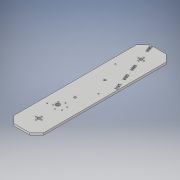
# Autodesk Inventor part: testPart_chassis2
Saved by Autodesk Inventor 2019 (Build 230136000, 136)
## iProperties
Created: 2019-09-17
Part Number: testPart_chassis2
Material: Generic
Document SubType Name: Modeling
Designer: shrey
Density: 1 g/cm^3
Appearance: Default
Author: shrey
Autodesk Inventor part; units mm, degrees
ref_plane "YZ Plane" through (0, 0, 0) normal (1, 0, 0) x (0, 1, 0)
ref_plane "XZ Plane" through (0, 0, 0) normal (0, 1, 0) x (-1, 0, 0)
ref_plane "XY Plane" through (0, 0, 0) normal (0, 0, 1) x (1, 0, 0)
sketch "Sketch1" plane through (0, 0, 0) normal (0, 1, 0) x (-1, 0, 0)
  line L0 (-44.45, -203.2) -> (44.45, -203.2)
  line L1 (44.45, -203.2) -> (44.45, 203.2)
  line L2 (44.45, 203.2) -> (-44.45, 203.2)
  line L3 (-44.45, 203.2) -> (-44.45, -203.2)
  line L4 (-44.45, -203.2) -> (44.45, 203.2) construction
  line L5 (44.45, -203.2) -> (-44.45, 203.2) construction
  line L6 (0, 203.2) -> (0, -203.2) construction
  line L7 (0, 0) -> (44.45, 0) construction
  line L8 (0, -203.2) -> (0, 203.2) construction
  line L9 (0, 152.4) -> (7.112, 152.4) construction
  line L10 (0, -152.4) -> (0, -203.2) construction
  circle A0 centre (0, -152.4) radius 8 construction
  line L11 (0, 152.4) -> (-44.45, 152.4) construction
  line L12 (-44.45, 152.4) -> (-44.45, 88.9)
  line L13 (-44.45, 88.9) -> (0, 88.9) construction
  line L14 (0, 88.9) -> (0, 152.4) construction
  circle A1 centre (0, 88.9) radius 7.112 construction
  circle A2 centre (7.112, 88.9) radius 5.9944
  circle A3 centre (0, 88.9) radius 15.494 construction
  circle A4 centre (0, 104.394) radius 1.5
  circle A5 centre (0, 88.9) radius 15.494 construction
  circle A6 centre (-13.4182, 96.647) radius 1.5
  circle A7 centre (0, 88.9) radius 15.494 construction
  circle A8 centre (-13.4182, 81.153) radius 1.5
  circle A9 centre (0, 88.9) radius 15.494 construction
  circle A10 centre (0, 73.406) radius 1.5
  circle A11 centre (0, 88.9) radius 15.494 construction
  circle A12 centre (13.4182, 81.153) radius 1.5
  circle A13 centre (0, 88.9) radius 15.494 construction
  circle A14 centre (13.4182, 96.647) radius 1.5
  circle A15 centre (0, 152.4) radius 4
  circle A16 centre (0, 152.4) radius 8 construction
  circle A17 centre (0, 160.4) radius 1.85
  circle A18 centre (0, 152.4) radius 8 construction
  circle A19 centre (-8, 152.4) radius 1.85
  circle A20 centre (0, 152.4) radius 8 construction
  circle A21 centre (0, 144.4) radius 1.85
  circle A22 centre (0, 152.4) radius 8 construction
  circle A23 centre (8, 152.4) radius 1.85
  line L15 (-88.9, 44.45) -> (0, 44.45) construction
  line L16 (0, 44.45) -> (0, -44.45) construction
  line L17 (0, -44.45) -> (-88.9, -44.45) construction
  line L18 (-88.9, -44.45) -> (-88.9, 44.45) construction
  line L19 (-88.9, 44.45) -> (0, -44.45) construction
  line L20 (0, 44.45) -> (-88.9, -44.45) construction
  circle A24 centre (0, 44.45) radius 2.9766
  circle A25 centre (0, -44.45) radius 2.9766
  line L21 (44.45, -203.2) -> (25.4, -203.2)
  line L22 (25.4, -203.2) -> (25.4, -101.6) construction
  line L23 (25.4, -101.6) -> (44.45, -101.6) construction
  line L24 (44.45, -101.6) -> (44.45, -203.2)
  circle A26 centre (25.9021, -101.6) radius 1.5875
  circle A27 centre (25.9021, 101.6) radius 1.5875
  line L25 (-44.45, 0) -> (-22.225, 0)
  line L26 (-44.45, -17.5714) -> (-25.4, -17.5714) construction
  line L27 (-25.4, -17.5714) -> (-25.4, 31.4423) construction
  line L28 (-25.4, 31.4423) -> (-44.45, 31.4423) construction
  line L29 (-44.45, 31.4423) -> (-44.45, -17.5714)
  circle A28 centre (-25.4, 0) radius 1.5875
  line L30 (-44.45, -203.2) -> (0, -203.2)
  line L31 (0, 0) -> (-44.45, 0)
  line L32 (-44.45, 0) -> (-44.45, -203.2)
  line L33 (-44.45, -203.2) -> (19.05, -203.2)
  line L34 (19.05, -203.2) -> (19.05, -25.4) construction
  line L35 (19.05, -25.4) -> (-44.45, -25.4) construction
  line L36 (-44.45, -25.4) -> (-44.45, -203.2)
  line L37 (19.05, -203.2) -> (-44.45, -25.4) construction
  line L38 (-44.45, -25.4) -> (-38.0428, -43.3402) construction
  line L39 (-30.3832, -55.3489) -> (-36.3634, -57.4842)
  line L40 (-36.3634, -57.4842) -> (-42.7694, -39.5436)
  line L41 (-42.7694, -39.5436) -> (-36.7892, -37.4083)
  line L42 (-36.7892, -37.4083) -> (-30.3832, -55.3489)
  line L43 (-41.2178, -33.8152) -> (-34.8678, -52.8652) construction
  line L44 (-34.8678, -33.8152) -> (-41.2178, -52.8652) construction
  line L45 (-23.549, -93.3646) -> (-29.955, -75.424)
  line L46 (-17.5688, -91.2293) -> (-23.549, -93.3646)
  line L47 (-23.9748, -73.2887) -> (-17.5688, -91.2293)
  line L48 (-29.955, -75.424) -> (-23.9748, -73.2887)
  line L49 (-10.7346, -129.245) -> (-17.1406, -111.3044)
  line L50 (-4.7544, -127.1096) -> (-10.7346, -129.245)
  line L51 (-11.1604, -109.169) -> (-4.7544, -127.1096)
  line L52 (-17.1406, -111.3044) -> (-11.1604, -109.169)
  line L53 (2.0798, -165.1253) -> (-4.3262, -147.1847)
  line L54 (8.06, -162.99) -> (2.0798, -165.1253)
  line L55 (1.654, -145.0494) -> (8.06, -162.99)
  line L56 (-4.3262, -147.1847) -> (1.654, -145.0494)
  line L57 (14.8942, -201.0057) -> (8.4882, -183.0651)
  line L58 (20.8744, -198.8704) -> (14.8942, -201.0057)
  line L59 (14.4684, -180.9298) -> (20.8744, -198.8704)
  line L60 (8.4882, -183.0651) -> (14.4684, -180.9298)
  circle A29 centre (0, -152.4) radius 4
  circle A30 centre (0, -160.4) radius 1.85
  circle A31 centre (-8, -152.4) radius 1.85
  circle A32 centre (0, -144.4) radius 1.85
  circle A33 centre (8, -152.4) radius 1.85
  dimension "d26" = 14.224
  dimension "d28" = 30.988
  dimension "d40" = 16
  dimension "d0" = 406.4
  dimension "d1" = 88.9
  dimension "d2" = 152.4
  dimension "d17" = 16
  dimension "d24" = 44.45
  dimension "d25" = 63.5
  dimension "d27" = 11.9888
  dimension "d29" = 3
  dimension "d32" = 360
  dimension "d39" = 8
  dimension "d41" = 3.7
  dimension "d44" = 360
  dimension "d63" = 88.9
  dimension "d64" = 5.9531
  dimension "d65" = 5.9531
  dimension "d71" = 101.6
  dimension "d72" = 19.05
  dimension "d73" = 3.175
  dimension "d74" = 19.05
  dimension "d75" = 3.175
  dimension "d81" = 177.8
  dimension "d82" = 63.5
  dimension "d83" = 19.05
  dimension "d84" = 6.35
  dimension "d85" = 19.05
  dimension "d88" = 38.1
  constraints: 122 end point, 23 centre point, 15 parallel, 10 midpoint, 9 coincident, 9 horizontal, 9 point on line, 9 symmetric about line, 7 perpendicular, 4 vertical alignment, 3 horizontal alignment, 1 collinear, 105 other
  measures "d0" distance of L0.end L1.end
  measures "d1" distance of L1.end L2.end
  measures "d2" distance of L7.start point (0, 152.4)
  measures "d17" diameter of A0
  measures "d24" distance of L9.start L11.end
  measures "d25" distance of L11.end L12.end
  measures "d27" diameter of A2
  measures "d29" diameter of A4
  measures "d39" diameter of A15
  measures "d41" diameter of A17
  measures "d63" distance of L17.end L15.start
  measures "d64" diameter of A24
  measures "d65" diameter of A25
  measures "d71" distance of L21.end L22.end
  measures "d72" distance of L22.end L23.end
  measures "d73" diameter of A26
  measures "d74" distance of L26.start L26.end
  measures "d75" diameter of A28
  measures "d81" distance of L33.end L34.end
  measures "d82" distance of L34.end L35.end
  measures "d83" distance of L35.end L38.end
  measures "d84" distance of L40.end L41.end
  measures "d85" distance of L39.end L40.end
  measures "d88" distance of L39.end L45.start
extrude "Extrusion8" add sketch "Sketch1" along normal blind 6.35 contours L3 L2 L1 L0 | L53 A30 A29 L56 A32 L55 L54
chamfer "Chamfer7" distance 20.32 angle 45 4 edges at (44.45, 3.175, 203.2) (-44.45, 3.175, 203.2) (44.45, 3.175, -203.2) (-44.45, 3.175, -203.2)
body "Solid8"
